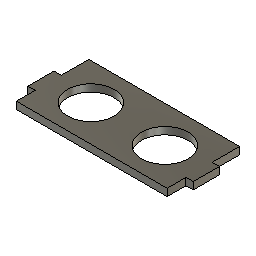
6thLessonUltrassonicSensorBase v2 (Autodesk Fusion 360 design; units mm, degrees)
Autodesk Fusion 360 part; units mm, degrees
sketch "Sketch1" plane through (0, 0, 0) normal (0, 0, 1) x (1, 0, 0)
  line L0 (15, 60) -> (67, 60)
  line L1 (67, 60) -> (67, 50.5)
  line L2 (15, 60) -> (15, 50.5)
  line L3 (67, 50.5) -> (69.5, 50.5)
  line L4 (15, 50.5) -> (12.5, 50.5)
  line L5 (69.5, 50.5) -> (69.5, 41.5)
  line L6 (12.5, 50.5) -> (12.5, 41.5)
  line L7 (69.5, 41.5) -> (67, 41.5)
  line L8 (12.5, 41.5) -> (15, 41.5)
  line L9 (67, 41.5) -> (67, 35)
  line L10 (15, 41.5) -> (15, 35)
  line L11 (67, 35) -> (15, 35)
  line L12 (15, 35) -> (15, 29) construction
  circle A0 centre (28.3, 47.4) radius 8
  line L13 (28.3, 47.4) -> (53.8, 47.4) construction
  circle A1 centre (53.8, 47.4) radius 8
  dimension "d1" = 52
  dimension "d2" = 9.5
  dimension "d3" = 9.5
  dimension "d4" = 2.5
  dimension "d5" = 2.5
  dimension "d6" = 9
  dimension "d7" = 9
  dimension "d8" = 2.5
  dimension "d9" = 2.5
  dimension "d10" = 6.5
  dimension "d11" = 6.5
  dimension "d12" = 16
  dimension "d13" = 12.4
  dimension "d14" = 15.8
  dimension "d15" = 25.5
  dimension "d16" = 16
  constraint horizontal L0
  constraint perpendicular L0 L1
  constraint perpendicular L0 L2
  constraint horizontal L3
  constraint horizontal L4
  constraint perpendicular L3 L5
  constraint perpendicular L4 L6
  constraint horizontal L7
  constraint horizontal L8
  constraint perpendicular L7 L9
  constraint perpendicular L8 L10
  constraint perpendicular L11 L12
  constraint coincident A0.centre L13.start
  constraint horizontal L13
  constraint coincident L13.end A1.centre
  measures "d1" distance of L0.start L0.end
  measures "d2" distance of L0.end L1.end
  measures "d3" distance of L0.start L2.end
  measures "d4" distance of L1.end L3.end
  measures "d5" distance of L2.end L4.end
  measures "d6" distance of L3.end L5.end
  measures "d7" distance of L4.end L6.end
  measures "d8" distance of L5.end L7.end
  measures "d9" distance of L6.end L8.end
  measures "d10" distance of L7.end L9.end
  measures "d11" distance of L8.end L10.end
  measures "d12" diameter of A0
  measures "d13" distance of L11 A0.centre
  measures "d14" distance of L6 A0.centre
  measures "d15" distance of A0.centre L13.end
  measures "d16" diameter of A1
extrude "Extrude1" add sketch "Sketch1" along normal blind 2.5
